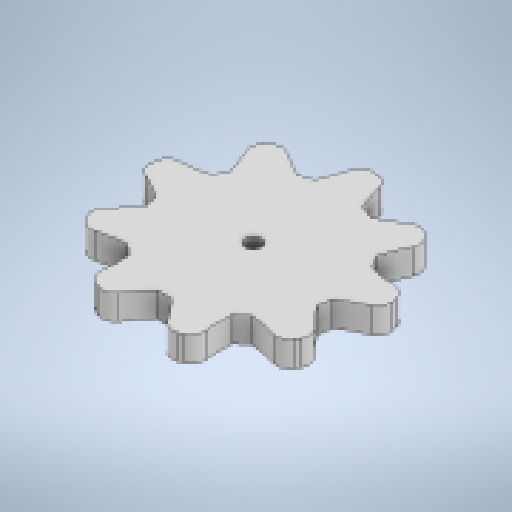
# Autodesk Inventor part: Motor Gear
Saved by Autodesk Inventor 2023 (Build 270158000, 158)
## iProperties
Created: 2023-02-22
Part Number: Motor Gear
Material: Generic
Document SubType Name: Modeling
Designer: cheng
Density: 1 g/cm^3
Appearance: Default
Author: cheng
Autodesk Inventor part; units mm, degrees
ref_plane "YZ Plane" through (0, 0, 0) normal (1, 0, 0) x (0, 1, 0)
ref_plane "XZ Plane" through (0, 0, 0) normal (0, 1, 0) x (-1, 0, 0)
ref_plane "XY Plane" through (0, 0, 0) normal (0, 0, 1) x (1, 0, 0)
sketch "Sketch1" plane through (0, 0, 0) normal (0, 1, 0) x (-1, 0, 0)
  circle A0 centre (0, 0) radius 55
  circle A1 centre (0, 0) radius 35
  line L0 (0, 0) -> (0, -55)
  circle A2 centre (0, 0) radius 3.175
  arc A3 (9.4265, -33.7067) -> (3.9925, -54.8549) centre (70.0543, -60.5571) ccw
  arc A4 (-3.9925, -54.8549) -> (-9.4265, -33.7067) centre (-70.0543, -60.5571) ccw
  arc A5 (28.8874, -19.7616) -> (38.3185, -39.455) centre (92.59, -1.3595) ccw
  arc A6 (32.2016, -44.5876) -> (14.4451, -31.8801) centre (-14.7393, -91.4195) ccw
  arc A7 (34.8315, 3.4302) -> (54.7148, -5.5936) centre (71.8019, 58.4743) ccw
  arc A8 (53.3282, -13.4573) -> (31.5577, -15.1364) centre (47.4723, -79.5056) ccw
  arc A9 (24.4776, 25.0169) -> (45.5095, 30.8851) centre (17.4169, 90.9473) ccw
  arc A10 (49.502, 23.9698) -> (33.9041, 8.6898) centre (87.4711, -30.3902) ccw
  arc A11 (2.6704, 34.898) -> (15.0098, 52.9123) centre (-45.1177, 80.8651) ccw
  arc A12 (22.5132, 50.1812) -> (20.3864, 28.4499) centre (86.5412, 32.9451) ccw
  arc A13 (-20.3864, 28.4499) -> (-22.5132, 50.1812) centre (-86.5412, 32.9451) ccw
  arc A14 (-15.0098, 52.9123) -> (-2.6704, 34.898) centre (45.1177, 80.8651) ccw
  arc A15 (-33.9041, 8.6898) -> (-49.502, 23.9698) centre (-87.4711, -30.3902) ccw
  arc A16 (-45.5095, 30.8851) -> (-24.4776, 25.0169) centre (-17.4169, 90.9473) ccw
  arc A17 (-31.5577, -15.1364) -> (-53.3282, -13.4573) centre (-47.4723, -79.5056) ccw
  arc A18 (-54.7148, -5.5936) -> (-34.8315, 3.4302) centre (-71.8019, 58.4743) ccw
  arc A19 (-14.4451, -31.8801) -> (-32.2016, -44.5876) centre (14.7393, -91.4195) ccw
  arc A20 (-38.3185, -39.455) -> (-28.8874, -19.7616) centre (-92.59, -1.3595) ccw
  circle A21 centre (0, 0) radius 48
  point P0 (14.4451, -31.8801)
  point P1 (32.2016, -44.5876)
  point P2 (38.3185, -39.455)
  point P3 (28.8874, -19.7616)
  point P4 (31.5577, -15.1364)
  point P5 (53.3282, -13.4573)
  point P6 (54.7148, -5.5936)
  point P7 (34.8315, 3.4302)
  point P8 (33.9041, 8.6898)
  point P9 (49.502, 23.9698)
  point P10 (45.5095, 30.8851)
  point P11 (24.4776, 25.0169)
  point P12 (20.3864, 28.4499)
  point P13 (22.5132, 50.1812)
  point P14 (15.0098, 52.9123)
  point P15 (2.6704, 34.898)
  point P16 (-2.6704, 34.898)
  point P17 (-15.0098, 52.9123)
  point P18 (-22.5132, 50.1812)
  point P19 (-20.3864, 28.4499)
  point P20 (-24.4776, 25.0169)
  point P21 (-45.5095, 30.8851)
  point P22 (-49.502, 23.9698)
  point P23 (-33.9041, 8.6898)
  point P24 (-34.8315, 3.4302)
  point P25 (-54.7148, -5.5936)
  point P26 (-53.3282, -13.4573)
  point P27 (-31.5577, -15.1364)
  point P28 (-28.8874, -19.7616)
  point P29 (-38.3185, -39.455)
  point P30 (-32.2016, -44.5876)
  point P31 (-14.4451, -31.8801)
  point P32 (-9.4265, -33.7067)
  point P33 (-3.9925, -54.8549)
  point P34 (-25.0848, 25.0848)
  point P35 (-9.1817, 34.2665)
  point P36 (9.1817, 34.2665)
  point P37 (25.0848, 25.0848)
  point P38 (34.2665, 9.1817)
  point P39 (34.2665, -9.1817)
  point P40 (25.0848, -25.0848)
  point P41 (9.1817, -34.2665)
  point P42 (26.8577, -39.7827)
  point P43 (34.5145, -33.3579)
  point P44 (46.146, -13.2115)
  point P45 (47.8817, -3.3681)
  point P46 (43.8421, 19.5415)
  point P47 (38.8445, 28.1976)
  point P48 (21.0239, 43.1508)
  point P49 (11.6315, 46.5694)
  point P50 (-11.6315, 46.5694)
  point P51 (-21.0239, 43.1508)
  point P52 (-38.8445, 28.1976)
  point P53 (-43.8421, 19.5415)
  point P54 (-47.8817, -3.3681)
  point P55 (-46.146, -13.2115)
  point P56 (-34.5145, -33.3579)
  point P57 (-26.8577, -39.7827)
  point P58 (-4.9976, -47.7391)
  point P59 (4.9976, -47.7391)
  dimension "d0" = 70
  dimension "d1" = 20
  dimension "d17" = 6.35
  dimension "d21" = 7.985
  dimension "d24" = 360
  dimension "d30" = 18.853
  dimension "d31" = 7
  dimension "d33" = 96
  constraints: 38 point on circle, 21 centre point, 4 coincident, 3 symmetric about line, 2 end point, 1 vertical, 77 other
  measures "d17" diameter of A2
  measures "d21" distance of A4.start A0.end
  measures "d30" distance of A4.end A3.start
  measures "d31" radial gap between concentric circles of A0 A21
  measures "d33" diameter of A21
extrude "Extrusion1" add sketch "Sketch1" along normal blind 10 contours A10 A1 A9 A21 | A21 A8 A1 A7 | A1 | A12 A1 A11 A21 | A21 A6 A1 A5 | A14 A1 A13 A21 | A21 L0 A1 A3 | A21 A4 A1 L0 | A16 A1 A15 A21 | A21 A20 A1 A19 | A18 A1 A17 A21
fillet "Fillet1" radius 5 18 edges at (-11.6315, 5, 46.5694) (-21.0239, 5, 43.1508) (11.6315, 5, 46.5694) (21.0239, 5, 43.1508) (38.8445, 5, 28.1976) (43.8421, 5, 19.5415) (47.8817, 5, -3.3681) (-38.8445, 5, 28.1976) (-43.8421, 5, 19.5415) (-47.8817, 5, -3.3681) (-46.146, 5, -13.2115) (-34.5145, 5, -33.3579) (46.146, 5, -13.2115) (34.5145, 5, -33.3579) (26.8577, 5, -39.7827) (4.9976, 5, -47.7391) (-4.9976, 5, -47.7391) (-26.8577, 5, -39.7827)
body "Solid1"
